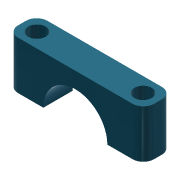
# Autodesk Inventor part: Motorhalterung_oben
Saved by Autodesk Inventor 2018.3 (Build 223284000, 284)
## iProperties
Created: 2016-11-17
Part Number: Motorhalterung_oben
Material: ABS-Kunststoff
Document SubType Name: Modeling
Designer: stud_brinkmann
Density: 1.06 g/cm^3
Appearance: Glatt - weiß
Mass: 0.904023 g
Surface Area: 9.15629 cm^2
Volume: 0.852852 cm^3
Author: stud_brinkmann
Autodesk Inventor part; units mm, degrees
ref_plane "YZ Plane" through (0, 0, 0) normal (1, 0, 0) x (0, 1, 0)
ref_plane "XZ Plane" through (0, 0, 0) normal (0, 1, 0) x (-1, 0, 0)
ref_plane "XY Plane" through (0, 0, 0) normal (0, 0, 1) x (1, 0, 0)
sketch "Skizze1" plane through (0, 0, 0) normal (0, 1, 0) x (-1, 0, 0)
  line L0 (0, 0) -> (-25.5, 0)
  line L1 (-25.5, 0) -> (-25.5, 9)
  line L2 (-25.5, 9) -> (0, 9)
  line L3 (0, 9) -> (0, 0)
  dimension "d0" = 25.5
  dimension "d1" = 9
  constraints: 8 end point, 2 parallel, 1 horizontal, 1 perpendicular
  measures "d0" distance of L1.end L2.end
  measures "d1" distance of L2.end L0.start
extrude "Extrusion1" add sketch "Skizze1" along normal blind 5.5
sketch "Skizze2" plane through (0, 0, 0) normal (0, -1, 0) x (1, 0, 0)
  line L0 (25.5, 0) -> (0, 0) projected
  arc A0 (18.75, 0) -> (6.75, 0) centre (12.75, 0) ccw
  dimension "d4" = 12
  constraints: 2 point on circle, 2 point on line, 1 centre point, 1 midpoint
  measures "d4" diameter of A0
extrude "Extrusion2" cut sketch "Skizze2" against normal through all
sketch "Skizze5" plane through (0, 0, 9) normal (0, 0, 1) x (1, 0, 0)
  line L0 (0, 0) -> (0, 5.5) construction
  line L1 (0, 2.75) -> (25.5934, 2.75) construction
  line L2 (25.5, 0) -> (0, 0) construction
  line L3 (12.75, 0) -> (12.75, 5.5) construction
  line L4 (0, 5.5) -> (25.5, 5.5) construction
  point P0 (2.8, 2.75)
  point P1 (22.7, 2.75)
  dimension "d33" = 2.8
  constraints: 4 end point, 3 midpoint, 1 horizontal, 1 point on line, 1 symmetric about line
  measures "d33" distance from line of L0 point (2.8, 2.75)
hole "Bohrung4" at (2.8, 2.75, 9) at (22.7, 2.75, 9) direction (0, 0, -1) diameter 3.3 end through all
fillet "Rundung1" radius 2 4 edges at (25.5, 0, 4.5) (25.5, 5.5, 4.5) (0, 0, 4.5) (0, 5.5, 4.5)
